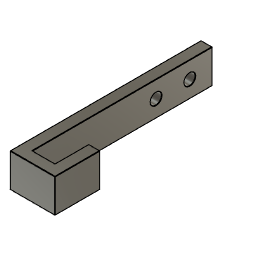
Key hook (Autodesk Fusion 360 design; units mm, degrees)
Autodesk Fusion 360 part; units mm, degrees
sketch "Sketch1" plane through (0, 0, 0) normal (0, 0, 1) x (1, 0, 0)
  line L0 (0, 0) -> (15, 0)
  line L1 (15, 0) -> (15, 5)
  line L2 (15, 5) -> (0, 5)
  line L3 (0, 5) -> (0, 0)
  line L4 (0, 5) -> (5, 5)
  line L5 (5, 5) -> (5, 85)
  line L6 (5, 85) -> (0, 85)
  line L7 (0, 85) -> (0, 5)
  line L8 (15, 0) -> (20, 0)
  line L9 (20, 0) -> (20, 20)
  line L10 (20, 20) -> (15, 20)
  line L11 (15, 20) -> (15, 0)
  dimension "d1" = 15
  dimension "d2" = 5
  dimension "d3" = 80
  dimension "d4" = 20
  constraint horizontal L0
  constraint vertical L1
  constraint horizontal L2
  constraint vertical L3
  constraint coincident L0.start L3.end
  constraint horizontal L4
  constraint vertical L5
  constraint horizontal L6
  constraint vertical L7
  constraint horizontal L8
  constraint vertical L9
  constraint horizontal L10
  constraint vertical L11
  measures "d1" distance of L0.start L0.end
  measures "d2" distance of L0.start L2.end
  measures "d3" distance of L2.end L6.end
  measures "d4" distance of L0.end L10.end
extrude "Extrude1" add sketch "Sketch1" along normal blind 15
sketch "Sketch2" plane through (0, 0, 0) normal (-1, 0, 0) x (0, -1, 0)
  line L0 (-85, 0) -> (0, 0)
  line L1 (0, 0) -> (0, 15)
  line L2 (0, 15) -> (-85, 15)
  line L3 (-85, 15) -> (-85, 0)
  circle A0 centre (-75, 7.5) radius 2.5
  circle A1 centre (-60, 7.5) radius 2.5
  dimension "d8" = 5
  dimension "d9" = 5
  dimension "d10" = 7.5
  dimension "d11" = 7.5
  dimension "d12" = 10
  dimension "d13" = 15
  measures "d8" diameter of A0
  measures "d9" diameter of A1
  measures "d10" distance of L2 A0.centre
  measures "d11" distance of L2 A1.centre
  measures "d12" distance of L3 A0.centre
  measures "d13" distance of A0.centre A1.centre
extrude "Extrude2" cut sketch "Sketch2" against normal blind 5 contours A0 | A1
fillet "Fillet1" radius 0.15 3 edges at (20, 20, 7.5) (20, 10, 15) (20, 10, 0)
fillet "Fillet2" radius 0.15 2 edges at (19.9561, 19.9561, 0.0439) (17.425, 20, 0)
fillet "Fillet3" radius 0.15 5 edges at (19.9561, 19.9561, 14.9561) (17.425, 20, 15) (15, 12.425, 0) (15, 19.9561, 0.0439) (15, 20, 7.575)
fillet "Fillet4" radius 0.15 4 edges at (15.0439, 19.9561, 14.9561) (15, 12.425, 15) (10, 5, 15) (5, 45, 15)
fillet "Fillet5" radius 0.15 7 edges at (9.925, 0, 0) (19.9561, 0, 0.0439) (20, 0, 7.5) (19.9561, 0, 14.9561) (9.925, 0, 15) (0, 0, 7.5) (0, 42.5, 15)
fillet "Fillet6" radius 0.15 5 edges at (5, 85, 7.425) (4.9561, 85, 14.9561) (2.5, 85, 15) (0.0439, 85, 14.9561) (0, 85, 7.425)
fillet "Fillet7" radius 0.15 6 edges at (5, 44.925, 0) (4.9561, 84.9561, 0) (2.5, 85, 0) (0.0439, 84.9561, 0) (0, 42.5, 0) (0.0439, 0.0439, 0.0439)
fillet "Fillet8" radius 0.15 1 edges at (10, 5, 0)
fillet "Fillet9" radius 0.15 2 edges at (5, 62.3308, 6.596) (5, 77.3308, 6.596)
